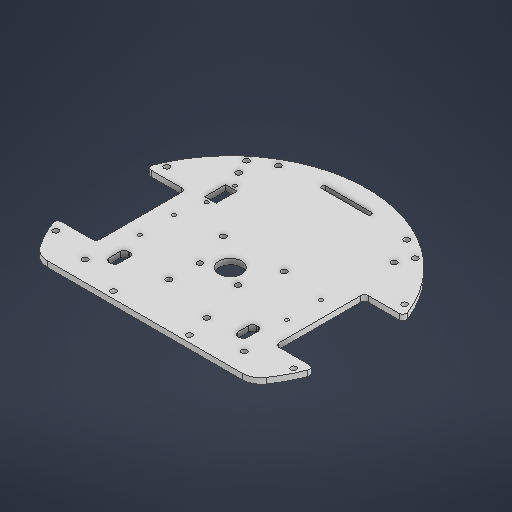
# Autodesk Inventor part: base_chasis_v6
Saved by Autodesk Inventor 2025.2 (Build 292293000, 293)
## iProperties
Created: 2025-03-12
Part Number: base_chasis_v6
Material: Generic
Document SubType Name: Modeling
Designer: cdavi
Density: 1 g/cm^3
Appearance: Default
Author: cdavi
Autodesk Inventor part; units mm, degrees
ref_plane "YZ Plane" through (0, 0, 0) normal (1, 0, 0) x (0, 1, 0)
ref_plane "XZ Plane" through (0, 0, 0) normal (0, 1, 0) x (-1, 0, 0)
ref_plane "XY Plane" through (0, 0, 0) normal (0, 0, 1) x (1, 0, 0)
sketch "Sketch1" plane through (0, 0, 0) normal (0, 1, 0) x (-1, 0, 0)
  line L0 (51.1762, 45) -> (-51.1762, 45)
  line L1 (12, -62.25) -> (-12, -62.25)
  line L2 (-12, -60) -> (12, -60)
  circle A0 centre (0, 0) radius 6
  circle A1 centre (-44.3523, -52.8571) radius 1.5
  circle A2 centre (-41.7906, 34.5) radius 1.5
  circle A3 centre (-62.5352, -29.1607) radius 1.5
  circle A4 centre (62.5352, -29.1607) radius 1.5
  circle A5 centre (-20, 41.5) radius 1.5
  circle A6 centre (41.7906, 34.5) radius 1.5
  circle A7 centre (20, 41.5) radius 1.5
  circle A8 centre (44.3523, -52.8571) radius 1.5
  arc A9 (12, -62.25) -> (12, -60) centre (12, -61.125) ccw
  arc A10 (-12, -60) -> (-12, -62.25) centre (-12, -61.125) ccw
  circle A11 centre (0, 0) radius 69 construction
  line L3 (0, 0) -> (0, 45)
  arc A12 (-59.4304, 40.6452) -> (59.4304, 40.6452) centre (0, 0) ccw
  arc A13 (-51.1762, 45) -> (-59.4304, 40.6452) centre (-51.1762, 35) ccw
  arc A14 (59.4304, 40.6452) -> (51.1762, 45) centre (51.1762, 35) ccw
  line L4 (0, 0) -> (-72, 0)
  line L5 (0, 0) -> (62.5352, -29.1607) construction
  line L6 (0, 0) -> (69, 0)
  line L7 (0, 0) -> (41.7906, 34.5) construction
  line L8 (47.057, 23.5) -> (68.057, 23.5)
  line L9 (68.057, 23.5) -> (68.057, -23.5)
  line L10 (68.057, -23.5) -> (47.057, -23.5)
  line L11 (47.057, -23.5) -> (47.057, 23.5)
  line L12 (47.057, 23.5) -> (68.057, -23.5) construction
  line L13 (68.057, 23.5) -> (47.057, -23.5) construction
  circle A15 centre (38.657, -9) radius 1
  circle A16 centre (38.657, 9) radius 1
  circle A17 centre (16, -12.35) radius 1.5
  circle A18 centre (33.75, -59) radius 1.5
  circle A19 centre (-16, -12.35) radius 1.5
  circle A20 centre (-33.75, -59) radius 1.5
  line L14 (-47.057, 23.5) -> (-68.057, 23.5)
  line L15 (-68.057, 23.5) -> (-68.057, -23.5)
  line L16 (-68.057, -23.5) -> (-47.057, -23.5)
  line L17 (-47.057, -23.5) -> (-47.057, 23.5)
  circle A21 centre (-38.657, -9) radius 1
  circle A22 centre (-38.657, 9) radius 1
  line L18 (39, -25.5) -> (33, -25.5)
  line L19 (33, -25.5) -> (33, -36.5)
  line L20 (33, -36.5) -> (39, -36.5)
  line L21 (39, -36.5) -> (39, -25.5)
  circle A23 centre (36, -38.5) radius 1
  line L22 (39, -31) -> (33, -31)
  circle A24 centre (36, -23.5) radius 1
  circle A25 centre (40.817, -45.3318) radius 1.5
  circle A26 centre (-41.7906, 34.5) radius 1.5
  circle A27 centre (-40.817, -45.3318) radius 1.5
  line L23 (41.7906, 34.5) -> (41.7906, 39.5)
  line L24 (41.7906, 39.5) -> (60.1976, 39.5) construction
  line L25 (0, 0) -> (44.3523, -52.8571) construction
  circle A28 centre (62.5352, 29.1607) radius 1.5
  circle A29 centre (-62.5352, 29.1607) radius 1.5
  line L26 (40.817, -45.3318) -> (0, 0) construction
  line L27 (0, 0) -> (62.5352, 29.1607) construction
  circle A30 centre (10, 6) radius 1.5
  circle A31 centre (-10, 6) radius 1.5
  line L28 (33.2906, 29.5) -> (34.2906, 29.5)
  line L29 (36.2906, 27.5) -> (36.2906, 21.5)
  line L30 (34.2906, 19.5) -> (33.2906, 19.5)
  line L31 (31.2906, 21.5) -> (31.2906, 27.5)
  arc A32 (34.2906, 19.5) -> (36.2906, 21.5) centre (34.2906, 21.5) ccw
  arc A33 (31.2906, 21.5) -> (33.2906, 19.5) centre (33.2906, 21.5) ccw
  arc A34 (33.2906, 29.5) -> (31.2906, 27.5) centre (33.2906, 27.5) ccw
  arc A35 (36.2906, 27.5) -> (34.2906, 29.5) centre (34.2906, 27.5) ccw
  line L32 (0, 0) -> (-41.7906, 34.5) construction
  line L33 (-33.2906, 29.5) -> (-34.2906, 29.5)
  line L34 (-36.2906, 27.5) -> (-36.2906, 21.5)
  line L35 (-34.2906, 19.5) -> (-33.2906, 19.5)
  line L36 (-31.2906, 21.5) -> (-31.2906, 27.5)
  arc A36 (-36.2906, 21.5) -> (-34.2906, 19.5) centre (-34.2906, 21.5) ccw
  arc A37 (-33.2906, 19.5) -> (-31.2906, 21.5) centre (-33.2906, 21.5) ccw
  arc A38 (-31.2906, 27.5) -> (-33.2906, 29.5) centre (-33.2906, 27.5) ccw
  arc A39 (-34.2906, 29.5) -> (-36.2906, 27.5) centre (-34.2906, 27.5) ccw
  circle A40 centre (0, 0) radius 54.1913
  point P0 (-5.9883, -61.0615)
  point P1 (57.557, 0)
  point P2 (68.057, 23.5)
  point P3 (-68.057, 23.5)
  point P4 (-68.057, -23.5)
  point P5 (0, 34.5)
  point P6 (36, -36.5)
  point P7 (55.8424, 43.8445)
  point P8 (0, -6)
  point P9 (31.2906, 29.5)
  point P10 (31.2906, 19.5)
  point P11 (33.7906, 29.5)
  point P12 (-31.2906, 29.5)
  point P13 (-31.2906, 19.5)
  point P14 (-33.7906, 29.5)
  dimension "d12" = 12
  dimension "d398" = 108.3827
  dimension "d0" = 3
  dimension "d1" = 3
  dimension "d4" = 3
  dimension "d15" = 24
  dimension "d16" = 3
  dimension "d62" = 2.25
  dimension "d148" = 3.5
  dimension "d276" = 138
  dimension "d285" = 144
  dimension "d286" = 45
  dimension "d287" = 10
  dimension "d288" = 12
  dimension "d289" = 40
  dimension "d290" = 3.5
  dimension "d291" = 20
  dimension "d293" = 25
  dimension "d300" = 21
  dimension "d301" = 47
  dimension "d304" = 2
  dimension "d305" = 8.4
  dimension "d306" = 9
  dimension "d307" = 3
  dimension "d311" = 16
  dimension "d318" = 33.75
  dimension "d323" = 11
  dimension "d324" = 6
  dimension "d325" = 2
  dimension "d326" = 2
  dimension "d327" = 15
  dimension "d338" = 33
  dimension "d342" = 5
  dimension "d345" = 11
  dimension "d346" = 39.541
  dimension "d348" = 40
  dimension "d350" = 61
  dimension "d351" = 48
  dimension "d352" = 3
  dimension "d353" = 12.35
  dimension "d354" = 59
  dimension "d355" = 25
  dimension "d356" = 60
  dimension "d358" = 68.057
  dimension "d371" = 3
  dimension "d372" = 10
  dimension "d373" = 6
  dimension "d393" = 5
  dimension "d394" = 10
  dimension "d395" = 5
  dimension "d396" = 2
  dimension "d397" = 8
  constraints: 75 end point, 39 centre point, 36 point on circle, 30 symmetric about line, 13 tangent, 11 point on line, 8 horizontal, 8 midpoint, 7 coincident, 7 parallel, 6 equal radius, 5 perpendicular, 3 vertical alignment, 2 vertical, 1 horizontal alignment, 23 other
  measures "d0" diameter of A6
  measures "d1" diameter of A7
  measures "d4" diameter of A4
  measures "d15" distance of L1.end L1.start
  measures "d16" diameter of A8
  measures "d62" distance between parallel lines of L1 L2
  measures "d148" distance from line of L0 A7.centre
  measures "d276" diameter of A11
  measures "d285" diameter of A12
  measures "d286" distance from line of L0 point (0, 0)
  measures "d287" radius of A13
  measures "d288" horizontal distance of point (0, 0) A9.centre
  measures "d289" distance of A7.centre A5.centre
  measures "d290" distance from line of L0 A5.centre
  measures "d291" distance from line of L3 A7.centre
  measures "d293" angle of L6 L5
  measures "d300" distance of L9.end L10.end
  measures "d301" distance of L10.end L8.start
  measures "d304" diameter of A15
  measures "d305" distance from line of L11 A15.centre
  measures "d306" distance from line of L6 A15.centre
  measures "d307" diameter of A17
  measures "d311" horizontal distance of point (0, 0) A17.centre
  measures "d318" distance from line of L3 A18.centre
  measures "d323" distance of L18.end L19.end
  measures "d324" distance of L18.start L18.end
  measures "d325" distance from line of L10.end L18
  measures "d326" diameter of A23
  measures "d327" distance of A24.centre A23.centre
  measures "d338" distance between parallel lines of L3 L19
  measures "d342" distance of L7.end L23.end
  measures "d345" distance from line of L8 L7.end
  measures "d346" angle of L6 L7
  measures "d348" angle of L3 L25
  measures "d350" distance of L26.start L4.start
  measures "d351" angle of L6 L26
  measures "d352" diameter of A25
  measures "d353" vertical distance of point (0, 0) A17.centre
  measures "d354" distance from line of L6 A18.centre
  measures "d355" angle of L27 L6
  measures "d356" distance between parallel lines of L2 L4
  measures "d358" distance between parallel lines of L3 L15
  measures "d371" diameter of A30
  measures "d372" horizontal distance of A30.centre point (0, 0)
  measures "d373" vertical distance of point (0, 0) A30.centre
  measures "d393" distance between parallel lines of L31 L29
  measures "d394" distance of point (31.291, 19.5) point (31.291, 29.5)
  measures "d395" distance from line of L7.end L28
  measures "d396" radius of A32
  measures "d397" horizontal distance of L7.end point (33.791, 29.5)
extrude "Extrusion1" add sketch "Sketch1" along normal blind 3 contours A14 A12 L8 A40 A6 L0 | A40 A6 L8 L11 L6 A0 L3 L0 | L3 A0 L4 L17 L14 A40 A2 L0 | A40 A2 L14 A12 A13 L0 | A12 L16 A40 L10 | L6 L11 L10 A40 L16 L17 L4 A0
sketch "Sketch3" plane through (0, 3, 0) normal (0, 1, 0) x (1, 0, 0)
  line L0 (3, 0) -> (3, -20)
  circle A0 centre (-10.775, -21.6) radius 1.5
  line L1 (-51.1762, -45) -> (51.1762, -45) projected
  circle A1 centre (16.775, -29.1) radius 1.5
  point P0 (0, 0)
  dimension "d377" = 20
  dimension "d378" = 3
  dimension "d379" = 3
  dimension "d380" = 13.775
  dimension "d381" = 23.4
  dimension "d383" = 13.775
  dimension "d384" = 3
  dimension "d385" = 15.9
  constraints: 2 centre point, 2 end point, 1 vertical
  measures "d377" distance of L0.start L0.end
  measures "d378" distance from line of point (0, 0) L0
  measures "d379" diameter of A0
  measures "d380" distance from line of L0 A0.centre
  measures "d381" distance from line of A0.centre L1
  measures "d383" distance from line of A1.centre L0
  measures "d384" diameter of A1
  measures "d385" distance from line of A1.centre L1
fillet "Fillet1" radius 2 1 edges at (68.057, 1.5, 23.5)
fillet "Fillet2" radius 2 7 edges at (68.057, 1.5, -23.5) (-68.057, 1.5, -23.5) (-68.057, 1.5, 23.5) (-47.057, 1.5, -23.5) (-47.057, 1.5, 23.5) (47.057, 1.5, -23.5) (47.057, 1.5, 23.5)
sketch "Sketch2" plane through (0, 3, 0) normal (0, 1, 0) x (1, 0, 0)
  circle A0 centre (62.5352, 29.1607) radius 1.5 projected
  circle A1 centre (62.5352, -29.1607) radius 1.5 projected
  line L0 (62.5352, 29.1607) -> (62.5352, -29.1607)
  line L1 (62.5352, -29.1607) -> (62.5352, -30.3154)
  line L2 (62.5352, -27.1607) -> (61.0352, -27.1607)
  line L3 (-51.1762, -45) -> (51.1762, -45) projected
  line L4 (0, -45) -> (0, 72)
  arc A2 (67.0527, 26.2286) -> (-67.0527, 26.2286) centre (0, 0) ccw projected
  line L5 (59.4352, -31.1607) -> (59.4352, -27.1607)
  line L6 (59.4352, -27.1607) -> (61.0352, -27.1607)
  line L7 (62.5352, -27.1607) -> (62.5352, -30.3154)
  line L8 (59.4352, -31.1607) -> (59.4352, -32.6607)
  line L9 (59.4352, -32.6607) -> (62.5352, -32.6607)
  line L10 (62.5352, -32.6607) -> (62.5352, -30.3154)
  line L11 (62.5352, -29.1607) -> (59.4352, -29.1607)
  line L12 (-70, 0) -> (70, 0)
  line L13 (62.5352, 29.1607) -> (62.5352, 30.3154)
  line L14 (62.5352, 27.1607) -> (61.0352, 27.1607)
  line L15 (59.4352, 31.1607) -> (59.4352, 27.1607)
  line L16 (59.4352, 27.1607) -> (61.0352, 27.1607)
  line L17 (62.5352, 27.1607) -> (62.5352, 30.3154)
  line L18 (59.4352, 31.1607) -> (59.4352, 32.6607)
  line L19 (59.4352, 32.6607) -> (62.5352, 32.6607)
  line L20 (62.5352, 32.6607) -> (62.5352, 30.3154)
  line L21 (-62.5352, -27.1607) -> (-61.0352, -27.1607)
  line L22 (-59.4352, -31.1607) -> (-59.4352, -27.1607)
  line L23 (-59.4352, -27.1607) -> (-61.0352, -27.1607)
  line L24 (-62.5352, -27.1607) -> (-62.5352, -30.3154)
  line L25 (-59.4352, -31.1607) -> (-59.4352, -32.6607)
  line L26 (-59.4352, -32.6607) -> (-62.5352, -32.6607)
  line L27 (-62.5352, -32.6607) -> (-62.5352, -30.3154)
  line L28 (-62.5352, -29.1607) -> (-59.4352, -29.1607)
  line L29 (-59.4352, 32.6607) -> (-62.5352, 32.6607)
  line L30 (-59.4352, 31.1607) -> (-59.4352, 32.6607)
  line L31 (-59.4352, 31.1607) -> (-59.4352, 27.1607)
  line L32 (-59.4352, 27.1607) -> (-61.0352, 27.1607)
  line L33 (-62.5352, 27.1607) -> (-61.0352, 27.1607)
  line L34 (-62.5352, 32.6607) -> (-62.5352, 30.3154)
  line L35 (-62.5352, 29.1607) -> (-62.5352, 30.3154)
  line L36 (-62.5352, 27.1607) -> (-62.5352, 30.3154)
  line L37 (-62.5352, 29.1607) -> (-59.4352, 29.1607)
  line L38 (62.5352, 29.1607) -> (59.4352, 29.1607)
  point P0 (62.5352, 27.1607)
  point P1 (62.5352, 27.6607)
  point P2 (60.7226, 29.8154)
  point P3 (60.7226, -29.8154)
  point P4 (62.5352, -27.6607)
  point P5 (62.5352, -27.1607)
  point P6 (62.5352, 30.6607)
  point P7 (62.5352, -30.6607)
  dimension "d363" = 1.5
  dimension "d365" = 4
  dimension "d366" = 1.5
  dimension "d367" = 3.1
  dimension "d368" = 1.6
  constraints: 76 end point, 26 symmetric about line, 5 vertical, 4 parallel, 2 midpoint, 1 horizontal, 1 perpendicular, 1 point on circle, 1 point on line
  measures "d363" distance of L2.start L2.end
  measures "d365" distance of L5.start L5.end
  measures "d366" distance of L5.start L8.end
  measures "d367" distance of L8.end L9.end
  measures "d368" distance of L5.end L2.end
extrude "Extrusion2" [suppressed]
hole "Hole1" at (-10.775, 3, 21.6) at (16.775, 3, 29.1) direction (0, -1, 0) diameter 3 end through all
body "Solid1"
